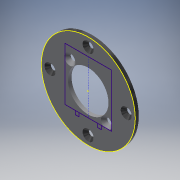
# Autodesk Inventor part: anschluss_daten
Saved by Autodesk Inventor 2018 (Build 220112000, 112)
## iProperties
Created: 2019-02-21
Part Number: anschluss_daten
Material: Generisch
Document SubType Name: Modeling
Designer: das RoboSAx OrgaTeam (pw)
Density: 1 g/cm^3
Appearance: Vorgabe
Project: RoboSAX Spielfeld
Author: das RoboSAx OrgaTeam (pw)
Autodesk Inventor part; units mm, degrees
ref_plane "YZ Plane" through (0, 0, 0) normal (1, 0, 0) x (0, 1, 0)
ref_plane "XZ Plane" through (0, 0, 0) normal (0, 1, 0) x (-1, 0, 0)
ref_plane "XY Plane" through (0, 0, 0) normal (0, 0, 1) x (1, 0, 0)
sketch "Skizze1" plane through (0, 0, 0) normal (0, 1, 0) x (-1, 0, 0)
  circle A0 centre (0, 0) radius 25.4
  dimension "d0" = 50.8
  constraints: 1 centre point, 1 coincident
  measures "d0" diameter of A0
extrude "Extrusion1" add sketch "Skizze1" along normal blind 2
sketch "Skizze2" plane through (0, 0, 0) normal (0, -1, 0) x (1, 0, 0)
  circle A0 centre (0, 0) radius 25.4 projected
  line L0 (-20.6475, 0) -> (0, 20.6475) construction
  line L1 (0, 20.6475) -> (20.6475, 0) construction
  line L2 (20.6475, 0) -> (0, -20.6475) construction
  line L3 (0, -20.6475) -> (-20.6475, 0) construction
  line L4 (0, 0) -> (10.3238, 10.3238) construction
  line L5 (0, 0) -> (-10.3238, 10.3238) construction
  circle A1 centre (0, 0) radius 25.4 construction
  line L6 (0, 0) -> (0, 25.4) construction
  point P0 (-20.6475, 0)
  point P1 (0, 20.6475)
  point P2 (20.6475, 0)
  dimension "d3" = 29.2
  dimension "d4" = 29.2
  dimension "d63" = 45
  constraints: 14 end point, 4 coincident, 3 perpendicular, 2 midpoint, 2 parallel, 1 vertical, 1 vertical alignment, 1 other
  measures "d3" distance of L0.start L0.end
  measures "d4" distance of L0.end L1.end
  measures "d63" angle of L6 L5
hole "Bohrung1" at (-20.6475, 0, 0) at (0, 0, 20.6475) at (20.6475, 0, 0) at (0, 0, -20.6475) direction (0, 1, 0) diameter 3 end through all countersink diameter 6 countersink angle 90
sketch "Skizze9" plane through (0, 0, 0) normal (0, -1, 0) x (1, 0, 0)
  circle A0 centre (0, 0) radius 25.4 projected
  circle A1 centre (0, 0) radius 11
  dimension "d53" = 22
  constraints: 1 centre point, 1 coincident
  measures "d53" diameter of A1
extrude "Extrusion7" cut sketch "Skizze9" against normal up to next contours A1
sketch "Skizze7" plane through (0, 0, 0) normal (0, -1, 0) x (1, 0, 0)
  circle A0 centre (0, 0) radius 25.4 construction
  line L0 (-9.9, 9.9) -> (9.9, 9.9) construction
  line L1 (9.9, 9.9) -> (9.9, -9.9) construction
  line L2 (9.9, -9.9) -> (-9.9, -9.9) construction
  line L3 (-9.9, -9.9) -> (-9.9, 9.9) construction
  line L4 (-9.9, 0) -> (9.9, 0) construction
  dimension "d42" = 19.8
  dimension "d43" = 19.8
  constraints: 11 end point, 3 coincident, 3 midpoint, 2 perpendicular, 1 horizontal, 1 parallel
  measures "d42" distance of L0.start L0.end
  measures "d43" distance of L0.end L1.end
hole "Bohrung3" at (-9.9, 0, 9.9) at (9.9, 0, -9.9) direction (0, 1, 0) diameter 3 end through all countersink diameter 6 countersink angle 90
sketch "Skizze10" plane through (0, 0, 0) normal (0, -1, 0) x (1, 0, 0)
  circle A0 centre (0, 0) radius 25.4 projected
  line L0 (-12.55, 16.2) -> (12.55, 16.2)
  line L1 (12.55, 16.2) -> (12.55, -12.5)
  line L2 (12.55, -12.5) -> (-12.55, -12.5)
  line L3 (-12.55, -12.5) -> (-12.55, 16.2)
  line L4 (0, 16.2) -> (0, -12.5) construction
  line L5 (-7, -12.5) -> (-5, -12.5) construction
  line L6 (-5, -12.5) -> (-5, -14.5)
  line L7 (-5, -14.5) -> (-7, -14.5)
  line L8 (-7, -14.5) -> (-7, -12.5)
  line L9 (5, -12.5) -> (7, -12.5) construction
  line L10 (7, -12.5) -> (7, -14.5)
  line L11 (7, -14.5) -> (5, -14.5)
  line L12 (5, -14.5) -> (5, -12.5)
  line L13 (-5, -12.5) -> (5, -12.5) construction
  dimension "d56" = 25.1
  dimension "d57" = 28.7
  dimension "d58" = 12.5
  dimension "d59" = 2
  dimension "d60" = 2
  dimension "d61" = 10
  dimension "d62" = 2
  constraints: 28 end point, 6 parallel, 4 point on line, 3 horizontal, 3 midpoint, 3 perpendicular, 1 collinear
  measures "d56" distance of L0.start L0.end
  measures "d57" distance of L2.end L0.start
  measures "d58" distance from line of point (0, 0) L2
  measures "d59" distance of L10.end L11.end
  measures "d60" distance of L6.end L7.end
  measures "d61" distance of L11.end L6.end
  measures "d62" distance of L9.end L10.end
